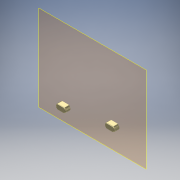
# Autodesk Inventor part: crystals
Saved by Autodesk Inventor 2016 (Build 200138000, 138)
## iProperties
Created: 2016-04-08
Part Number: crystals
Material: Generic
Document SubType Name: Modeling
Designer: Paschalis
Density: 1 g/cm^3
Appearance: Gold - Metal
Author: Paschalis
Autodesk Inventor part; units mm, degrees
ref_plane "YZ Plane" through (0, 0, 0) normal (1, 0, 0) x (0, 1, 0)
ref_plane "XZ Plane" through (0, 0, 0) normal (0, 1, 0) x (-1, 0, 0)
ref_plane "XY Plane" through (0, 0, 0) normal (0, 0, 1) x (1, 0, 0)
ref_plane "Work Plane1" through (27.775, 29.205, -0.1) normal (0, 0, 1) x (1, 0, 0)
sketch "Sketch1" plane through (27.775, 29.205, -0.1) normal (0, 0, 1) x (1, 0, 0)
  circle A0 centre (-30.19, -29.21) radius 0.405 projected
  circle A1 centre (-25.36, -29.21) radius 0.405 projected
  line L0 (-22.187, -26.411) -> (-33.363, -26.411) projected
  line L1 (-33.363, -26.411) -> (-33.363, -31.999) projected
  line L2 (-33.363, -31.999) -> (-22.187, -31.999) projected
  line L3 (-22.187, -31.999) -> (-22.187, -26.411) projected
  circle A2 centre (19.98, -20.95) radius 0.405 projected
  circle A3 centre (24.8, -20.95) radius 0.405 projected
  line L4 (16.802, -23.744) -> (27.978, -23.744) projected
  line L5 (27.978, -23.744) -> (27.978, -18.156) projected
  line L6 (27.978, -18.156) -> (16.802, -18.156) projected
  line L7 (16.802, -18.156) -> (16.802, -23.744) projected
  line L8 (-30.19, -29.21) -> (-25.36, -29.21) construction
  line L9 (-30.19, -26.421) -> (-25.36, -26.421)
  line L10 (-25.36, -31.999) -> (-30.19, -31.999)
  arc A4 (-30.19, -26.421) -> (-30.19, -31.999) centre (-30.19, -29.21) ccw
  arc A5 (-25.36, -31.999) -> (-25.36, -26.421) centre (-25.36, -29.21) ccw
  line L11 (19.98, -20.95) -> (24.8, -20.95) construction
  line L12 (19.98, -18.156) -> (24.8, -18.156)
  line L13 (24.8, -23.744) -> (19.98, -23.744)
  arc A6 (19.98, -18.156) -> (19.98, -23.744) centre (19.98, -20.95) ccw
  arc A7 (24.8, -23.744) -> (24.8, -18.156) centre (24.8, -20.95) ccw
  point P0 (-27.775, -29.205)
  point P1 (-27.775, -29.21)
  point P2 (22.39, -20.95)
  constraints: 16 end point, 8 point on circle, 8 tangent, 4 centre point, 3 parallel, 2 midpoint, 1 horizontal
extrude "Extrusion1" add sketch "Sketch1" along normal blind 5 contours A0 | A1 | L2 A4 L9 A5 | A2 | A3 | A6 L6 A7 L4
fillet "Fillet1" radius 1 8 edges at (0, 2.784, 4.9) (-5.204, -0.005, 4.9) (0, -2.794, 4.9) (5.204, -0.005, 4.9) (50.165, 11.049, 4.9) (44.961, 8.255, 4.9) (50.165, 5.461, 4.9) (55.369, 8.255, 4.9)
body "Solid1"
